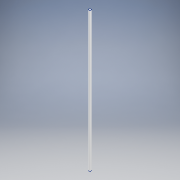
# Autodesk Inventor part: Y-Axis_Linear_Rod_1_4inx400mm_LM3038
Saved by Autodesk Inventor 2020.3 (Build 243373000, 373)
## iProperties
Created: 2020-05-30
Part Number: Y-Axis_Linear_Rod_1_4inx400mm_LM3038
Material: Aluminum 6061
Document SubType Name: Modeling
Designer: rah75
Density: 2.7 g/cm^3
Appearance: Aluminum - Flat
Author: rah75
Autodesk Inventor part; units mm, degrees
ref_plane "YZ Plane" through (0, 0, 0) normal (1, 0, 0) x (0, 1, 0)
ref_plane "XZ Plane" through (0, 0, 0) normal (0, 1, 0) x (-1, 0, 0)
ref_plane "XY Plane" through (0, 0, 0) normal (0, 0, 1) x (1, 0, 0)
sketch "Sketch1" plane through (0, 0, 0) normal (0, 1, 0) x (-1, 0, 0)
  circle A0 centre (0, 0) radius 3.175
  dimension "d0" = 6.35
  constraints: 1 centre point, 1 coincident
  measures "d0" diameter of A0
extrude "Extrusion1" add sketch "Sketch1" along normal mid plane 400
chamfer "Chamfer1" distance 0.5 angle 45 2 edges at (3.175, 200, 0) (3.175, -200, 0)
body "Solid1"
